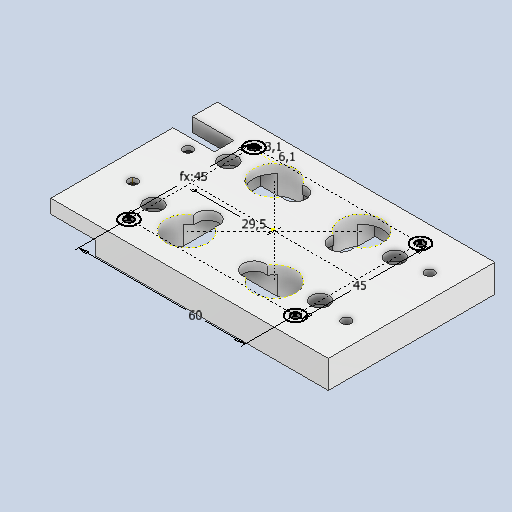
# Autodesk Inventor part: Oberteil_servoplatte
Saved by Autodesk Inventor 2024 (Build 280153000, 153)
## iProperties
Created: 2022-05-09
Part Number: Oberteil_servoplatte
Material: PBT-Kunststoff
Document SubType Name: Modeling
Designer: 123St
Density: 1.31 g/cm^3
Appearance: Glatt - Weiß
Mass: 50.4632 g
Surface Area: 180.173 cm^2
Volume: 38.5215 cm^3
Author: 123St
Autodesk Inventor part; units mm, degrees
ref_plane "YZ Plane" through (0, 0, 0) normal (1, 0, 0) x (0, 1, 0)
ref_plane "XZ Plane" through (0, 0, 0) normal (0, 1, 0) x (-1, 0, 0)
ref_plane "XY Plane" through (0, 0, 0) normal (0, 0, 1) x (1, 0, 0)
sketch "Skizze1" plane through (0, 0, 0) normal (0, 1, 0) x (-1, 0, 0)
  line L0 (50, -30) -> (-50, -30)
  line L1 (-50, -30) -> (-50, 30)
  line L2 (-50, 30) -> (50, 30)
  line L3 (50, 30) -> (50, -30)
  line L4 (-70, 0) -> (70, 0) projected
  line L5 (0, -42) -> (0, 42) projected
  point P0 (0, 0)
  dimension "d0" = 60
  dimension "d1" = 30
  dimension "d2" = 100
  dimension "d3" = 50
  constraints: 8 end point, 2 parallel, 1 horizontal, 1 perpendicular
  measures "d0" distance between parallel lines of L2 L0
  measures "d1" distance between parallel lines of L4 L0
  measures "d2" distance of L0.start L0.end
  measures "d3" distance between parallel lines of L5 L1
extrude "Extrusion1" add sketch "Skizze1" along normal blind 10
sketch "Skizze2" plane through (0, 10, 0) normal (0, 1, 0) x (1, 0, 0)
  circle A0 centre (-40.5, 10) radius 1.5
  circle A1 centre (-40.5, -10) radius 1.5
  circle A2 centre (41.5, -15) radius 1.5
  circle A3 centre (41.5, 15) radius 1.5
  line L0 (-50, 30) -> (-50, -30) construction
  line L1 (70, 0) -> (-70, 0) construction
  point P0 (0, 0)
  dimension "d6" = 20
  dimension "d9" = 30
  dimension "d12" = 9.5
  dimension "d13" = 10
  dimension "d14" = 15
  dimension "d59" = 3
  dimension "d60" = 3
  dimension "d61" = 3
  dimension "d62" = 3
  dimension "d96" = 82
  dimension "d97" = 82
  dimension "d98" = 9.5
  constraints: 4 centre point
  measures "d6" distance of A1.centre A0.centre
  measures "d9" distance of A3.centre A2.centre
  measures "d12" distance from line of L0 A0.centre
  measures "d13" distance from line of L1 A0.centre
  measures "d14" distance from line of L1 A3.centre
  measures "d59" diameter of A0
  measures "d60" diameter of A1
  measures "d61" diameter of A2
  measures "d62" diameter of A3
  measures "d96" horizontal distance of A0.centre A3.centre
  measures "d97" horizontal distance of A2.centre A1.centre
  measures "d98" distance from line of L0 A1.centre
extrude "Extrusion2" cut sketch "Skizze2" against normal blind 10
sketch "Skizze3" plane through (0, 0, 0) normal (0, -1, 0) x (1, 0, 0)
  circle A0 centre (16.25, -15.75) radius 7.5
  circle A1 centre (16.25, 15.75) radius 7.5
  circle A2 centre (-15.25, 15.75) radius 7.5
  circle A3 centre (-15.25, -15.75) radius 7.5
  line L0 (50, 30) -> (50, -30) projected
  circle A4 centre (41.5, -15) radius 1.5 projected
  line L1 (-70, 0) -> (70, 0) projected
  circle A5 centre (41.5, 15) radius 1.5 projected
  line L2 (16.25, 15.75) -> (-15.25, 15.75) construction
  line L3 (-15.25, 15.75) -> (-15.25, -15.75) construction
  point P0 (0, 0)
  dimension "d18" = 31.5
  dimension "d19" = 15
  dimension "d20" = 15
  dimension "d21" = 15
  dimension "d22" = 15
  dimension "d26" = 25.25
  dimension "d27" = 15.75
  dimension "d29" = 25.25
  dimension "d135" = 31.5
  dimension "d136" = 31.5
  constraints: 4 centre point, 4 end point, 1 horizontal, 1 vertical
  measures "d18" distance of A0.centre L2.start
  measures "d19" diameter of A0
  measures "d20" diameter of A3
  measures "d21" diameter of A2
  measures "d22" diameter of A1
  measures "d26" horizontal distance of A0.centre A4.centre
  measures "d27" distance from line of L1 A0.centre
  measures "d29" horizontal distance of A5.centre L2.start
  measures "d135" distance of L2.start L2.end
  measures "d136" distance of L2.end L3.end
extrude "Extrusion3" cut sketch "Skizze3" against normal blind 10 contours A0 | A1 | A2 | A3
sketch "Skizze4" plane through (0, 0, 0) normal (0, -1, 0) x (1, 0, 0)
  line L0 (-25.7656, -21.465) -> (7.0258, -21.465)
  line L1 (7.0258, -21.465) -> (7.0258, -10.035)
  line L2 (7.0258, -10.035) -> (-25.7656, -10.035)
  line L3 (-25.7656, -10.035) -> (-25.7656, -21.465)
  circle A0 centre (-15.25, -15.75) radius 7.5 projected
  line L4 (26.7656, 10.035) -> (-6.0258, 10.035)
  line L5 (-6.0258, 10.035) -> (-6.0258, 21.465)
  line L6 (-6.0258, 21.465) -> (26.7656, 21.465)
  line L7 (26.7656, 21.465) -> (26.7656, 10.035)
  line L8 (21.965, -26.2656) -> (10.535, -26.2656)
  line L9 (10.535, -26.2656) -> (10.535, 6.5258)
  line L10 (10.535, 6.5258) -> (21.965, 6.5258)
  line L11 (21.965, 6.5258) -> (21.965, -26.2656)
  line L12 (-20.965, 26.2656) -> (-9.535, 26.2656)
  line L13 (-9.535, 26.2656) -> (-9.535, -6.5258)
  line L14 (-9.535, -6.5258) -> (-20.965, -6.5258)
  line L15 (-20.965, -6.5258) -> (-20.965, 26.2656)
  circle A1 centre (16.25, -15.75) radius 7.5 projected
  circle A2 centre (16.25, 15.75) radius 7.5 projected
  circle A3 centre (-15.25, 15.75) radius 7.5 projected
  point P0 (0, 0)
  dimension "d63" = 11.43
  dimension "d64" = 32.7914
  dimension "d65" = 5.715
  dimension "d67" = 5.715
  dimension "d68" = 11.43
  dimension "d69" = 32.7914
  dimension "d70" = 5.715
  dimension "d71" = 11.43
  dimension "d72" = 32.7914
  dimension "d73" = 5.715
  dimension "d74" = 11.43
  dimension "d75" = 32.7914
  dimension "d153" = 22.2758
  dimension "d154" = 22.2758
  dimension "d155" = 22.2758
  dimension "d156" = 22.2758
  constraints: 32 end point, 8 parallel, 4 horizontal, 4 perpendicular
  measures "d63" distance of L2.end L0.start
  measures "d64" distance of L0.start L0.end
  measures "d65" distance from line of A0.centre L2
  measures "d67" distance from line of L9 A1.centre
  measures "d68" distance of L8.start L8.end
  measures "d69" distance of L10.end L8.start
  measures "d70" distance from line of L6 A2.centre
  measures "d71" distance of L6.end L4.start
  measures "d72" distance of L5.end L6.end
  measures "d73" distance from line of A3.centre L15
  measures "d74" distance of L12.start L12.end
  measures "d75" distance of L14.end L12.start
  measures "d153" distance from line of L14 A3.centre
  measures "d154" distance from line of L1 A0.centre
  measures "d155" distance from line of L10 A1.centre
  measures "d156" distance from line of L5 A2.centre
extrude "Extrusion4" cut sketch "Skizze4" against normal blind 6.8 contours L3 L2 A0 L0 | A0 L2 L0 | A0 L2 L1 L0 | L4 A2 L6 L7 | L4 A2 L6 | L4 L5 L6 A2 | L8 L9 A1 L11 | A1 L9 L11 | A1 L9 L10 L11 | L12 L13 A3 L15 | A3 L13 L15 | A3 L13 L14 L15
sketch "Skizze5" plane through (0, 0, 0) normal (0, -1, 0) x (1, 0, 0)
  arc A0 (21.965, -10.8932) -> (10.535, -10.8932) centre (16.25, -15.75) ccw projected
  circle A1 centre (16.25, -8.25) radius 4
  arc A2 (-10.3932, -21.465) -> (-10.3932, -10.035) centre (-15.25, -15.75) ccw projected
  circle A3 centre (-7.75, -15.75) radius 4
  circle A4 centre (9.0005, 15.75) radius 4
  arc A5 (-20.965, 10.8932) -> (-9.535, 10.8932) centre (-15.25, 15.75) ccw projected
  circle A6 centre (-15.25, 8.25) radius 4
  dimension "d79" = 8
  dimension "d80" = 8
  dimension "d81" = 8
  dimension "d82" = 8
  constraints: 4 centre point, 3 point on circle
  measures "d79" diameter of A1
  measures "d80" diameter of A3
  measures "d81" diameter of A6
  measures "d82" diameter of A4
extrude "Extrusion5" cut sketch "Skizze5" against normal blind 10
sketch "Skizze6" plane through (0, 0, 0) normal (0, -1, 0) x (1, 0, 0)
  line L0 (-33.9, -30) -> (-50, -30)
  line L1 (-50, -30) -> (-50, 30)
  line L2 (-50, 30) -> (-33.9, 30)
  line L3 (-33.9, 30) -> (-33.9, -30)
  line L4 (-50, -30) -> (-50, 30) projected
  line L5 (50, -30) -> (-50, -30) projected
  line L6 (-50, 30) -> (50, 30) projected
  point P0 (0, 0)
  dimension "d85" = 0
  dimension "d86" = 0
  dimension "d87" = 0
  dimension "d88" = 16.1
  constraints: 8 end point, 2 parallel, 1 horizontal, 1 perpendicular
  measures "d85" distance between parallel lines of L4 L1
  measures "d86" distance between parallel lines of L5 L0
  measures "d87" distance between parallel lines of L6 L2
  measures "d88" distance between parallel lines of L1 L3
extrude "Extrusion6" cut sketch "Skizze6" against normal blind 5
sketch "Skizze7" plane through (0, 5, 0) normal (0, -1, 0) x (1, 0, 0)
  line L0 (-50, -30) -> (-50, 30) projected
  line L1 (-50, -21) -> (-35, -21)
  line L2 (-35, -21) -> (-35, -14)
  line L3 (-35, -14) -> (-50, -14)
  line L4 (-50, -14) -> (-50, -21)
  line L5 (-33.9, -30) -> (-50, -30) projected
  point P0 (0, 0)
  point P1 (-50, -14)
  dimension "d91" = 9
  dimension "d92" = 7
  dimension "d93" = 15
  constraints: 8 end point, 2 parallel, 1 horizontal, 1 perpendicular, 1 point on line
  measures "d91" distance between parallel lines of L5 L1
  measures "d92" distance of L1.end L2.end
  measures "d93" distance of L2.end L3.end
extrude "Extrusion7" cut sketch "Skizze7" against normal blind 6
sketch "Skizze8" plane through (0, 10, 0) normal (0, -1, 0) x (1, 0, 0)
  circle A0 centre (30.5, -13.5) radius 1.5 construction
  circle A1 centre (30.5, 13.5) radius 1.5 construction
  circle A2 centre (-29.5, 13.5) radius 1.5 construction
  circle A3 centre (-29.5, -13.5) radius 1.5 construction
  line L0 (50, -30) -> (-33.9, -30) projected
  line L1 (50, 30) -> (50, -30) projected
  line L2 (-33.9, 30) -> (50, 30) projected
  line L3 (-33.9, 30) -> (-33.9, -30) projected
  line L4 (30.5, -13.5) -> (-29.5, -13.5) construction
  line L5 (30.5, 13.5) -> (-29.5, 13.5) construction
  line L6 (-29.5, 13.5) -> (-29.5, -13.5) construction
  circle A4 centre (30.5, 22.5) radius 3.25 construction
  circle A5 centre (30.5, -22.5) radius 3.25 construction
  line L7 (30.5, 22.5) -> (30.5, -22.5) construction
  circle A6 centre (-29.5, 22.5) radius 3.25 construction
  circle A7 centre (-29.5, -22.5) radius 3.25 construction
  line L8 (-29.5, 22.5) -> (-29.5, -22.5) construction
  line L9 (30.5, 13.5) -> (30.5, -13.5) construction
  point P0 (0, 0)
  dimension "d103" = 3
  dimension "d104" = 3
  dimension "d105" = 16.5
  dimension "d106" = 16.5
  dimension "d109" = 3
  dimension "d110" = 3
  constraints: 12 end point, 5 coincident, 4 centre point, 3 vertical, 2 collinear, 2 horizontal, 1 perpendicular
  measures "d103" diameter of A1
  measures "d104" diameter of A0
  measures "d105" distance from line of L0 L4.end
  measures "d106" distance from line of L2 A2.centre
  measures "d109" diameter of A3
  measures "d110" diameter of A2
hole "Bohrung1" at (30.5, 10, 13.5) at (-29.5, 10, 13.5) at (30.5, 10, -13.5) at (-29.5, 10, -13.5) direction (0, -1, 0) diameter 3.4 end through all counterbore diameter 6.5 counterbore depth 3.4 clearance for "Inbusschraube DIN EN ISO 4762" size "M3" standard "DIN"
sketch "Skizze9" plane through (0, 10, 0) normal (0, 1, 0) x (1, 0, 0)
  line L0 (30.5, 22.5) -> (30.5, -22.5) construction
  line L1 (-29.5, -22.5) -> (-29.5, 22.5) construction
  circle A0 centre (-29.5, 22.5) radius 3.05
  circle A1 centre (-29.5, -22.5) radius 3.05
  circle A2 centre (30.5, 22.5) radius 3.05
  circle A3 centre (30.5, -22.5) radius 3.05
  circle A4 centre (-29.5, 22.5) radius 1.55
  circle A5 centre (30.5, 22.5) radius 1.55
  circle A6 centre (-29.5, -22.5) radius 1.55
  circle A7 centre (30.5, -22.5) radius 1.55
  line L2 (-29.5, 0) -> (30.5, 0) construction
  line L3 (-29.5, -22.5) -> (30.5, -22.5) construction
  line L4 (-20.1068, 21.465) -> (-25.7656, 21.465) construction
  line L5 (30.5, 22.5) -> (-29.5, 22.5) construction
  point P0 (0, 0)
  dimension "d164" = 6.1
  dimension "d168" = 3.1
  dimension "d178" = 45
  dimension "d179" = 45
  dimension "d180" = 60
  dimension "d182" = 29.5
  constraints: 10 end point, 8 centre point, 8 coincident, 6 equal radius, 2 midpoint, 2 vertical, 1 horizontal, 1 point on line
  measures "d164" diameter of A0
  measures "d168" diameter of A4
  measures "d178" distance of L0.start L0.end
  measures "d179" distance of L1.start L1.end
  measures "d180" distance of L0.end L1.start
  measures "d182" distance from line of point (0, 0) L1
extrude "Extrusion9" cut sketch "Skizze9" along normal blind 8 from surface at -10 contours A0 | A1 | A2 | A3 | A4 | A5 | A6 | A7
extrude "Extrusion12" cut sketch "Skizze9" against normal through all contours A4 | A5 | A6 | A7
ref_plane "Arbeitsebene1" through (-40.5, 10, 10) normal (-1, 0, 0) x (0, -1, 0)
ref_plane "Arbeitsebene2" through (-15.25, 0, 15.75) normal (-1, 0, 0) x (0, 1, 0)
sketch "Skizze12" plane through (0, 5, 0) normal (0, -1, 0) x (1, 0, 0)
  circle A0 centre (-40.5, 10) radius 1.5 construction
  circle A1 centre (-40.5, -10) radius 1.5 construction
  point P0 (0, 0)
  constraints: 2 coincident
sketch "Skizze13" plane through (0, 0, 0) normal (0, -1, 0) x (1, 0, 0)
  circle A0 centre (41.5, 15) radius 1.5 construction
  circle A1 centre (41.5, -15) radius 1.5 construction
  point P0 (0, 0)
  constraints: 2 coincident
hole "Bohrung2" at (-40.5, 5, 10) at (-40.5, 5, -10) direction (0, 1, 0) diameter 3.4 end through all counterbore diameter 6.5 counterbore depth 3.4 clearance for "Inbusschraube DIN EN ISO 4762" size "M3" standard "DIN"
hole "Bohrung3" at (41.5, 0, 15) at (41.5, 0, -15) direction (0, 1, 0) diameter 3.4 end through all counterbore diameter 6.5 counterbore depth 3.4 clearance for "Inbusschraube DIN EN ISO 4762" size "M3" standard "DIN"
thicken "Verdickung1" operation add thickness 0.2 both sides no extend neighbours yes toward (1, 0, 0) faces at (-9.535, 4.5333, 22.4931) (-13.345, 2.2667, 26.2656) (-20.965, 2.2667, 22.4931) (-20.965, 2.2667, -0.7195) (-9.535, 4.5333, 5.0868) (-17.155, 2.2667, -6.5258) (-6.0258, 2.2667, 17.655) (-0.2195, 4.5333, 21.465) (24.8793, 2.2667, 21.465) (26.7656, 2.2667, 13.845) (24.8793, 2.2667, 10.035) (5.5868, 4.5333, 10.035) (18.155, 4.5333, 6.5258) (10.535, 2.2667, 0.7195) (10.535, 2.2667, -22.4931) (1.2195, 2.2667, -10.035) (-21.9931, 4.5333, -10.035) (-25.7656, 2.2667, -13.845) (7.0258, 2.2667, -17.655) (21.965, 4.5333, -5.0868) (21.965, 4.5333, -22.4931) (-23.8793, 4.5333, -21.465) (1.2195, 2.2667, -21.465) (14.345, 2.2667, -26.2656)
sketch "Skizze15" plane through (0, 10, 0) normal (0, 1, 0) x (1, 0, 0)
  arc A0 (-19.1052, -9.3167) -> (-11.3948, -9.3167) centre (-15.25, -15.75) ccw construction
  arc A1 (-8.8167, 19.6052) -> (-8.8167, 11.8948) centre (-15.25, 15.75) ccw construction
  arc A2 (9.8492, -19.6589) -> (9.8492, -11.8411) centre (16.25, -15.75) ccw construction
  arc A3 (20.1052, 9.3167) -> (12.3948, 9.3167) centre (16.25, 15.75) ccw construction
  line L0 (-15.25, -15.75) -> (16.25, 15.75) construction
  line L1 (16.25, -15.75) -> (-15.25, 15.75) construction
  point P0 (0, 0)
  point P1 (0.5, 0)
  constraints: 4 end point, 1 midpoint
equation "\"d1\" = 0.5 * d0"
equation "\"d3\" = 0.5 * d2"
equation "\"d18\" = d135"
equation "\"d26\" = d29"
equation "\"d27\" = 0.5 * d18"
equation "\"d136\" = d135"
equation "\"d63\" = d74"
equation "\"d64\" = d75"
equation "\"d65\" = d73"
equation "\"d67\" = d73"
equation "\"d68\" = d74"
equation "\"d69\" = d75"
equation "\"d70\" = d73"
equation "\"d71\" = d74"
equation "\"d72\" = d75"
equation "\"d73\" = Side2MotorAxis_Dist"
equation "\"d74\" = Motor_width"
equation "\"d75\" = TotalWidth"
equation "\"d153\" = FarEdge2MainAxis"
equation "\"d154\" = d153"
equation "\"d155\" = d153"
equation "\"d156\" = d153"
equation "\"d106\" = d105"
equation "\"Side2MotorAxis_Dist\" = 5.715"
equation "\"Motor_width\" = 11.43"
equation "\"TotalWidth\" = 32.7914"
equation "\"FarEdge2MainAxis\" = 22.2758"
